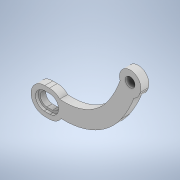
# Autodesk Inventor part: Part7
Saved by Autodesk Inventor 2020.3 (Build 243373000, 373)
## iProperties
Created: 2019-09-27
Part Number: Part7
Material: Generic
Document SubType Name: Modeling
Designer: Horváth Patrik
Density: 1 g/cm^3
Appearance: Default
Author: Horváth Patrik
Autodesk Inventor part; units mm, degrees
ref_plane "YZ Plane" through (0, 0, 0) normal (1, 0, 0) x (0, 1, 0)
ref_plane "XZ Plane" through (0, 0, 0) normal (0, 1, 0) x (-1, 0, 0)
ref_plane "XY Plane" through (0, 0, 0) normal (0, 0, 1) x (1, 0, 0)
sketch "Sketch1" plane through (0, 0, 0) normal (0, 0, 1) x (1, 0, 0)
  circle A0 centre (31, 22) radius 1.25
  circle A1 centre (31, 22) radius 3
  arc A2 (0, 0) -> (31, 22) centre (-0.1128, 32.9998) ccw construction
  arc A3 (0.0103, -3) -> (33.8284, 21) centre (-0.1128, 32.9998) ccw
  arc A4 (-0.0103, 3) -> (28.1716, 23) centre (-0.1128, 32.9998) ccw
  arc A5 (-0.0103, 3) -> (0.0103, -3) centre (0, 0) ccw
  arc A6 (33.8284, 21) -> (28.1716, 23) centre (31, 22) ccw
  point P0 (41.5332, 21.1583)
  point P1 (35.8668, 23.1312)
  point P2 (33.8284, 21)
  point P3 (28.1716, 23)
  dimension "d1" = 30
  dimension "d21" = 6
  dimension "d22" = 2.5
  dimension "d23" = 31
  dimension "d24" = 22
  constraints: 10 point on circle, 7 centre point, 4 tangent, 2 coincident, 1 concentric
  measures "d1" radius of A4
  measures "d21" radial gap between concentric circles of A3 A4
  measures "d22" diameter of A0
  measures "d23" horizontal distance of point (0, 0) A0.centre
  measures "d24" vertical distance of point (0, 0) A0.centre
extrude "Extrusion1" add sketch "Sketch1" along normal blind 3
sketch "Sketch3" plane through (0, 0, 3) normal (0, 0, 1) x (1, 0, 0)
  arc A0 (-1, 0.0117) -> (1, 0.0186) centre (-0.1128, 32.9998) ccw construction
  arc A1 (-1.1344, -4.9865) -> (1.1686, -4.9786) centre (-0.1128, 32.9998) ccw
  arc A2 (-0.8656, 5.0099) -> (0.8314, 5.0157) centre (-0.1128, 32.9998) ccw
  arc A3 (-0.8656, 5.0099) -> (-1.1344, -4.9865) centre (-1, 0.0117) ccw
  arc A4 (1.1686, -4.9786) -> (0.8314, 5.0157) centre (1, 0.0186) ccw
  arc A5 (0.0103, -3) -> (33.8284, 21) centre (-0.1128, 32.9998) ccw projected
  point P0 (0, 0)
  dimension "d31" = 10
  dimension "d32" = 1
  dimension "d33" = 1
  constraints: 11 point on circle, 5 centre point, 4 tangent, 1 concentric
  measures "d31" radial gap between concentric circles of A1 A2
  measures "d32" horizontal distance of point (0, 0) A0.start
  measures "d33" horizontal distance of A0.end point (0, 0)
extrude "Extrusion3" add sketch "Sketch3" against normal blind 3
sketch "Sketch4" plane through (0, 0, 3) normal (0, 0, -1) x (1, 0, 0)
  arc A0 (-1.1344, 4.9865) -> (-0.8656, -5.0099) centre (-1, -0.0117) ccw projected
  arc A1 (1.1686, 4.9786) -> (-1.1344, 4.9865) centre (-0.1128, -32.9998) ccw projected
  arc A2 (0.8314, -5.0157) -> (-0.8656, -5.0099) centre (-0.1128, -32.9998) ccw projected
  arc A3 (1, -0.0186) -> (-1, -0.0117) centre (-0.1128, -32.9998) ccw construction
  arc A4 (1.0843, 2.48) -> (-1.0672, 2.4874) centre (-0.1128, -32.9998) ccw
  arc A5 (0.9157, -2.5172) -> (-0.9328, -2.5108) centre (-0.1128, -32.9998) ccw
  arc A6 (0.9157, -2.5172) -> (1.0843, 2.48) centre (1, -0.0186) ccw
  arc A7 (-1.0672, 2.4874) -> (-0.9328, -2.5108) centre (-1, -0.0117) ccw
  arc A8 (28.1716, -23) -> (4.6946, -3.3875) centre (-0.1128, -32.9998) ccw projected
  arc A9 (28.1716, -23) -> (33.8284, -21) centre (31, -22) ccw projected
  arc A10 (33.8284, -21) -> (5.2614, 2.5968) centre (-0.1128, -32.9998) ccw projected
  arc A11 (5.2614, 2.5968) -> (1.1686, 4.9786) centre (1, -0.0186) ccw projected
  arc A12 (0.8314, -5.0157) -> (4.6946, -3.3875) centre (1, -0.0186) ccw projected
  arc A13 (0.8887, -3.3167) -> (-0.9113, -3.3105) centre (-0.1128, -32.9998) ccw
  arc A14 (0.8887, -3.3167) -> (1.1113, 3.2795) centre (1, -0.0186) ccw
  arc A15 (1.1113, 3.2795) -> (-1.0887, 3.2871) centre (-0.1128, -32.9998) ccw
  arc A16 (-1.0887, 3.2871) -> (-0.9113, -3.3105) centre (-1, -0.0117) ccw
  point P0 (0, 0)
  dimension "d43" = 5
  dimension "d52" = 0.8
  constraints: 18 point on circle, 9 centre point, 4 tangent, 2 coincident, 1 concentric, 3 other
  measures "d43" radial gap between concentric circles of A4 A5
  measures "d52" radial gap between concentric circles of A5 A13
extrude "Extrusion4" cut sketch "Sketch4" along normal through all contours A6 A5 A7 A4
sketch "Sketch5" plane through (0, 0, 3) normal (0, 0, 1) x (1, 0, 0)
  circle A0 centre (31, 22) radius 1.25 projected
  arc A1 (0, 0) -> (31, 22) centre (-0.1128, 32.9998) ccw construction
  arc A2 (34.7535, 20.6174) -> (27.2465, 23.3826) centre (31, 22) ccw
  arc A3 (26.9479, 22.5719) -> (34.4549, 19.8068) centre (30.7014, 21.1893) ccw
  line L0 (30.0441, 21.4413) -> (31.2665, 20.9727)
  line L1 (32.5586, 21.449) -> (29.5201, 22.5232)
  line L2 (26.9479, 22.5719) -> (27.2465, 23.3826)
  line L3 (34.4549, 19.8068) -> (34.7535, 20.6174)
  circle A4 centre (31, 22) radius 1.8
  dimension "d44" = 8
  dimension "d46" = 1.5
  dimension "d47" = 3.6
  constraints: 8 end point, 5 point on circle, 4 tangent, 3 centre point, 2 coincident, 2 line through centre, 2 point on line, 1 equal radius
  measures "d44" diameter of A2
  measures "d46" angle of L1 L0
  measures "d47" diameter of A4
extrude "Extrusion5" cut sketch "Sketch5" against normal up to surface (3 mm away) contours A4
extrude "Extrusion6" add sketch "Sketch5" against normal up to surface (3 mm away) contours L3 A3 L2 A2
extrude "Extrusion7" cut sketch "Sketch4" along normal blind 1 contours A13 A16 A15 A14
sketch "Sketch6" plane through (0, 0, 0) normal (0, 0, -1) x (-1, 0, 0)
  circle A0 centre (-31, 22) radius 1.8 projected
  arc A1 (-32.4154, 17.5752) -> (-5.2614, -2.5968) centre (0.1128, 32.9998) ccw projected
  arc A2 (-5.2614, -2.5968) -> (-1.1686, -4.9786) centre (-1, 0.0186) ccw projected
  arc A3 (-1.1686, -4.9786) -> (1.1344, -4.9865) centre (0.1128, 32.9998) ccw projected
  arc A4 (1.1344, -4.9865) -> (0.8656, 5.0099) centre (1, 0.0117) ccw projected
  arc A5 (-0.8314, 5.0157) -> (0.8656, 5.0099) centre (0.1128, 32.9998) ccw projected
  arc A6 (-0.8314, 5.0157) -> (-4.6946, 3.3875) centre (-1, 0.0186) ccw projected
  arc A7 (-26.899, 19.9475) -> (-4.6946, 3.3875) centre (0.1128, 32.9998) ccw projected
  arc A8 (-26.899, 19.9475) -> (-26.9479, 22.5719) centre (-30.7014, 21.1893) ccw projected
  line L0 (-26.9479, 22.5719) -> (-27.2465, 23.3826) projected
  arc A9 (-27.2465, 23.3826) -> (-34.7535, 20.6174) centre (-31, 22) ccw projected
  line L1 (-34.7535, 20.6174) -> (-34.4549, 19.8068) projected
  arc A10 (-34.4549, 19.8068) -> (-32.4154, 17.5752) centre (-30.7014, 21.1893) ccw projected
  arc A11 (-1.0843, -2.48) -> (1.0672, -2.4874) centre (0.1128, 32.9998) ccw projected
  arc A12 (-0.9157, 2.5172) -> (-1.0843, -2.48) centre (-1, 0.0186) ccw projected
  arc A13 (-0.9157, 2.5172) -> (0.9328, 2.5108) centre (0.1128, 32.9998) ccw projected
  arc A14 (1.0672, -2.4874) -> (0.9328, 2.5108) centre (1, 0.0117) ccw projected
  arc A15 (-27.2465, 23.3826) -> (-34.7535, 20.6174) centre (-31, 22) ccw projected
  arc A16 (-27.2315, 20.6591) -> (-27.2465, 23.3826) centre (-31, 22) ccw
  arc A17 (-26.899, 19.9475) -> (-4.6946, 3.3875) centre (0.1128, 32.9998) ccw projected
  arc A18 (-27.2315, 20.6591) -> (-26.899, 19.9475) centre (0.1128, 32.9998) ccw
  arc A19 (-26.899, 19.9475) -> (-4.6946, 3.3875) centre (0.1128, 32.9998) ccw projected
  point P0 (0, 0)
  constraints: 6 point on circle, 3 concentric, 2 centre point
extrude "Extrusion8" cut sketch "Sketch6" against normal up to surface (3 mm away) contours L0 A8 A18 A16
sketch "Sketch7" plane through (0, 0, 3) normal (0, 0, 1) x (1, 0, 0)
  arc A0 (34.7535, 20.6174) -> (27.2315, 20.6591) centre (31, 22) ccw projected
  arc A1 (4.6946, 3.3875) -> (27.2315, 20.6591) centre (-0.1128, 32.9998) ccw projected
  arc A2 (4.6946, 3.3875) -> (0.8314, 5.0157) centre (1, 0.0186) ccw projected
  arc A3 (-0.8656, 5.0099) -> (0.8314, 5.0157) centre (-0.1128, 32.9998) ccw projected
  arc A4 (-0.8656, 5.0099) -> (-1.1344, -4.9865) centre (-1, 0.0117) ccw projected
  arc A5 (-1.1344, -4.9865) -> (1.1686, -4.9786) centre (-0.1128, 32.9998) ccw projected
  arc A6 (1.1686, -4.9786) -> (5.2614, -2.5968) centre (1, 0.0186) ccw projected
  arc A7 (5.2614, -2.5968) -> (32.4154, 17.5752) centre (-0.1128, 32.9998) ccw projected
  arc A8 (32.4154, 17.5752) -> (34.4549, 19.8068) centre (30.7014, 21.1893) ccw projected
  line L0 (34.4549, 19.8068) -> (34.7535, 20.6174) projected
  circle A9 centre (31, 22) radius 1.8 projected
  arc A10 (-1.0887, -3.2871) -> (1.1113, -3.2795) centre (-0.1128, 32.9998) ccw projected
  arc A11 (-0.9113, 3.3105) -> (-1.0887, -3.2871) centre (-1, 0.0117) ccw projected
  arc A12 (-0.9113, 3.3105) -> (0.8887, 3.3167) centre (-0.1128, 32.9998) ccw projected
  arc A13 (1.1113, -3.2795) -> (0.8887, 3.3167) centre (1, 0.0186) ccw projected
  arc A14 (5.2614, -2.5968) -> (32.4154, 17.5752) centre (-0.1128, 32.9998) ccw projected
  arc A15 (5.2614, -2.5968) -> (27.6993, 8.5472) centre (6.5569, 22.9556) ccw
  arc A16 (27.6993, 8.5472) -> (32.4154, 17.5752) centre (-8.4143, 33.1583) ccw
  arc A17 (4.6946, 3.3875) -> (22.8001, 11.886) centre (6.5569, 22.9556) ccw
  arc A18 (34.7535, 20.6174) -> (27.2315, 20.6591) centre (31, 22) ccw projected
  arc A19 (22.8001, 11.886) -> (27.2315, 20.6591) centre (-8.4143, 33.1583) ccw
  line L1 (5.2614, -2.5968) -> (4.6946, 3.3875)
  line L2 (4.6946, 3.3875) -> (2.1704, 20.8058)
  line L3 (2.1704, 20.8058) -> (15.0141, 27.6003)
  line L4 (15.0141, 27.6003) -> (27.2315, 20.6591)
  point P0 (0, 0)
  constraints: 9 point on circle, 8 end point, 4 centre point, 2 concentric, 2 tangent, 1 point on line
extrude "Extrusion9" cut sketch "Sketch7" against normal up to surface (3 mm away) contours A19 A17 A1 | A1 L2 L3 L4
extrude "Extrusion10" add sketch "Sketch7" against normal up to surface (3 mm away) contours A16 A15 A7
body "Solid1"
